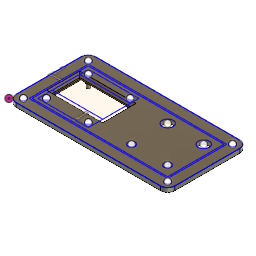
kkClave_Front_Panel v1 (Autodesk Fusion 360 design; units mm, degrees)
Autodesk Fusion 360 part; units mm, degrees
sketch "Sketch2" plane through (0, 0, 0) normal (0, 0, 1) x (1, 0, 0)
  line L0 (5, 0) -> (105, 0)
  line L1 (110, 5) -> (110, 50)
  line L2 (105, 55) -> (5, 55)
  line L3 (0, 50) -> (0, 5)
  line L4 (10, 45) -> (45, 45)
  line L5 (45, 45) -> (45, 10)
  line L6 (45, 10) -> (10, 10)
  line L7 (10, 10) -> (10, 45)
  circle A0 centre (95, 40) radius 3.75
  circle A1 centre (70, 40) radius 3.75
  circle A2 centre (95, 15) radius 2.5
  circle A3 centre (70, 15) radius 2.5
  line L8 (10, 39) -> (45, 39)
  line L9 (45, 39) -> (45, 20)
  line L10 (45, 20) -> (10, 20)
  line L11 (10, 20) -> (10, 39)
  circle A4 centre (13, 42) radius 1.25
  circle A5 centre (42, 42) radius 1.25
  circle A6 centre (13, 13) radius 1.25
  circle A7 centre (42, 13) radius 1.25
  circle A8 centre (13, 42) radius 2
  circle A9 centre (42, 42) radius 2
  circle A10 centre (13, 13) radius 2
  circle A11 centre (42, 13) radius 2
  circle A12 centre (5, 50) radius 2
  circle A13 centre (105, 50) radius 2
  circle A14 centre (5, 5) radius 2
  circle A15 centre (105, 5) radius 2
  arc A16 (5, 55) -> (0, 50) centre (5, 50) ccw
  arc A17 (110, 50) -> (105, 55) centre (105, 50) ccw
  arc A18 (105, 0) -> (110, 5) centre (105, 5) ccw
  arc A19 (0, 5) -> (5, 0) centre (5, 5) ccw
  line L12 (8, 47) -> (102, 47)
  line L13 (102, 47) -> (102, 8)
  line L14 (102, 8) -> (8, 8)
  line L15 (8, 8) -> (8, 47)
  line L16 (7, 48) -> (103, 48)
  line L17 (103, 48) -> (103, 7)
  line L18 (103, 7) -> (7, 7)
  line L19 (7, 7) -> (7, 48)
  dimension "d3" = 7.5
  dimension "d4" = 20
  dimension "d5" = 10
  dimension "d6" = -25
  dimension "d7" = -25
  dimension "d8" = 5
  dimension "d9" = 20
  dimension "d10" = 10
  dimension "d11" = -25
  dimension "d12" = 0
  dimension "d13" = 2.5
  dimension "d14" = 20
  dimension "d15" = 20
  dimension "d16" = 29
  dimension "d17" = -29
  dimension "d18" = 4
  dimension "d19" = 20
  dimension "d20" = 20
  dimension "d21" = 29
  dimension "d22" = -29
  dimension "d23" = 4
  dimension "d24" = 20
  dimension "d25" = 20
  dimension "d26" = 100
  dimension "d27" = -45
  dimension "d28" = 5
  constraint horizontal L0
  constraint vertical L1
  constraint horizontal L2
  constraint vertical L3
  constraint horizontal L4
  constraint vertical L5
  constraint horizontal L6
  constraint vertical L7
  constraint horizontal L8
  constraint vertical L9
  constraint horizontal L10
  constraint vertical L11
  constraint coincident L5 L9.end
  constraint coincident L7 L8.start
  constraint concentric A4 A8
  constraint tangent L2 A16
  constraint tangent L3 A16
  constraint tangent L1 A17
  constraint tangent L2 A17
  constraint equal A16 A17
  constraint tangent L0 A18
  constraint tangent L1 A18
  constraint equal A16 A18
  constraint tangent L0 A19
  constraint tangent L3 A19
  constraint equal A16 A19
  constraint horizontal L12
  constraint vertical L13
  constraint horizontal L14
  constraint vertical L15
  constraint horizontal L16
  constraint vertical L17
  constraint horizontal L18
  constraint vertical L19
  measures "d3" diameter of A0
  measures "d8" diameter of A2
  measures "d13" diameter of A4
  measures "d18" diameter of A8
  measures "d23" diameter of A12
  measures "d28" radius of A16
extrude "Extrude1" add sketch "Sketch2" against normal blind 3 contours L0 L1 L2 L3 A16 A17 A18 A19 | L4 L5 L7 L8 | L5 L6 L7 L10 | L12 L13 L14 L15 makes body 1 at (71.066, 1.3774, 0) makes body 2 at (60.2764, 24.5895, 0)
extrude "Extrude2" add sketch "Sketch2" against normal blind 6 contours L16 L17 L18 L19 bodies 1 2
extrude "Extrude3" add sketch "Sketch2" against normal blind 4.5 contours A8 | A9 | A10 | A11 bodies 1
extrude "Extrude4" add sketch "Sketch2" against normal blind 8 contours A4 | A5 | A6 | A7 bodies 1
chamfer "Chamfer1" distance 2 angle 45 4 edges at (27.5, 20, 0) (27.5, 39, 0) (45, 29.5, 0) (10, 29.5, 0) on bodies 1
